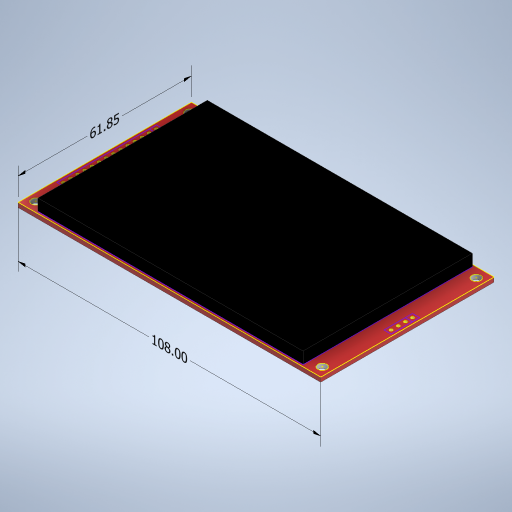
# Autodesk Inventor part: ILI9488
Saved by Autodesk Inventor 2024 (Build 280153000, 153)
## iProperties
Created: 2024-01-05
Part Number: ILI9488
Material: Genérico
Document SubType Name: Modeling
Designer: sergi
Density: 1 g/cm^3
Appearance: Valor por defecto
Author: sergi
Autodesk Inventor part; units mm, degrees
ref_plane "YZ Plane" through (0, 0, 0) normal (1, 0, 0) x (0, 1, 0)
ref_plane "XZ Plane" through (0, 0, 0) normal (0, 1, 0) x (-1, 0, 0)
ref_plane "XY Plane" through (0, 0, 0) normal (0, 0, 1) x (1, 0, 0)
sketch "Boceto1" plane through (0, 0, 0) normal (0, 1, 0) x (-1, 0, 0)
  line L0 (-54, 30.925) -> (54, 30.925)
  line L1 (54, 30.925) -> (54, -30.925)
  line L2 (54, -30.925) -> (-54, -30.925)
  line L3 (-54, -30.925) -> (-54, 30.925)
  line L4 (-54, 30.925) -> (54, -30.925) construction
  line L5 (54, 30.925) -> (-54, -30.925) construction
  line L6 (54, -30.925) -> (54, -29.075)
  circle A0 centre (-51.1, -27.475) radius 1.6
  circle A1 centre (51.1, -27.475) radius 1.6
  circle A2 centre (51.1, 27.475) radius 1.6
  circle A3 centre (-51.1, 27.475) radius 1.6
  line L7 (54, 30.925) -> (54, 29.075)
  line L8 (-50.7696, -29.075) -> (-51.1, -29.075)
  line L9 (-50.7696, 29.075) -> (-51.1, 29.075)
  line L10 (51.1, 29.075) -> (50.7696, 29.075)
  point P0 (0, 0)
  dimension "d4" = 3.2
  dimension "d6" = 3.2
  dimension "d7" = 3.2
  dimension "d0" = 108
  dimension "d1" = 61.85
  dimension "d5" = 3.2
  constraints: 22 end point, 6 horizontal, 5 point on line, 4 perpendicular, 3 vertical alignment, 2 midpoint, 2 parallel, 1 centre point, 1 tangent, 6 other
  measures "d0" distance of L1.end L2.end
  measures "d1" distance of L0.end L1.end
  measures "d5" diameter of A1
extrude "Extrusión1" add sketch "Boceto1" along normal blind 1.65
sketch "Boceto2" plane through (0, 1.65, 0) normal (0, 1, 0) x (1, 0, 0)
  line L0 (54, -30.925) -> (54, 30.925) projected
  line L1 (54, 30.925) -> (-54, 30.925) projected
  line L2 (-54, 30.925) -> (-54, -30.925) projected
  line L3 (-54, -30.925) -> (54, -30.925) projected
  circle A0 centre (51.1, 27.475) radius 1.6 projected
  circle A1 centre (-51.1, 27.475) radius 1.6 projected
  circle A2 centre (-51.1, -27.475) radius 1.6 projected
  circle A3 centre (51.1, -27.475) radius 1.6 projected
  line L4 (54, 30.925) -> (54, 5.075)
  line L5 (54, -30.925) -> (54, 30.925) projected
  line L6 (54, 5.075) -> (53.25, 5.075)
  line L7 (53.25, 5.075) -> (50.71, 5.075)
  line L8 (50.71, 5.075) -> (50.71, -5.085)
  line L9 (50.71, -5.085) -> (53.25, -5.085)
  line L10 (53.25, -5.085) -> (53.25, 5.075)
  line L11 (51.98, 5.075) -> (51.98, -5.085)
  line L12 (51.98, 5.075) -> (51.98, 3.805)
  line L13 (51.98, 3.805) -> (51.98, 1.265)
  line L14 (51.98, 1.265) -> (51.98, -1.275)
  line L15 (51.98, -1.275) -> (51.98, -3.815)
  circle A4 centre (51.98, 3.805) radius 0.5
  circle A5 centre (51.98, 1.265) radius 0.5
  circle A6 centre (51.98, -1.275) radius 0.5
  circle A7 centre (51.98, -3.815) radius 0.5
  line L16 (-54, 30.925) -> (-53.25, 30.925)
  line L17 (54, 30.925) -> (-54, 30.925) projected
  line L18 (-53.25, 30.925) -> (-53.25, 17.675)
  line L19 (-53.25, 17.675) -> (-50.71, 17.675)
  line L20 (-50.71, 17.675) -> (-50.71, -17.885)
  line L21 (-50.71, -17.885) -> (-53.25, -17.885)
  line L22 (-53.25, -17.885) -> (-53.25, 17.675)
  line L23 (-51.98, 17.675) -> (-51.98, 16.405)
  circle A8 centre (-51.98, 16.405) radius 0.5
  line L24 (-51.98, 16.405) -> (-51.98, 13.851)
  line L25 (-51.98, 15.121) -> (-51.98, 13.851)
  circle A9 centre (-51.98, 13.851) radius 0.5
  line L26 (-51.98, 13.851) -> (-51.98, 11.297)
  line L27 (-51.98, 12.567) -> (-51.98, 11.297)
  circle A10 centre (-51.98, 11.297) radius 0.5
  line L28 (-51.98, 11.297) -> (-51.98, 8.743)
  line L29 (-51.98, 8.743) -> (-51.98, 6.189)
  circle A11 centre (-51.98, 8.743) radius 0.5
  line L30 (-51.98, 6.189) -> (-51.98, 3.635)
  circle A12 centre (-51.98, 6.189) radius 0.5
  line L31 (-51.98, 3.635) -> (-51.98, 1.081)
  circle A13 centre (-51.98, 3.635) radius 0.5
  line L32 (-51.98, 1.081) -> (-51.98, -1.473)
  circle A14 centre (-51.98, 1.081) radius 0.5
  line L33 (-51.98, -1.473) -> (-51.98, -4.027)
  circle A15 centre (-51.98, -1.473) radius 0.5
  line L34 (-51.98, -4.027) -> (-51.98, -6.581)
  circle A16 centre (-51.98, -4.027) radius 0.5
  line L35 (-51.98, -6.581) -> (-51.98, -9.135)
  circle A17 centre (-51.98, -6.581) radius 0.5
  line L36 (-51.98, -9.135) -> (-51.98, -11.689)
  circle A18 centre (-51.98, -9.135) radius 0.5
  line L37 (-51.98, -11.689) -> (-51.98, -14.243)
  circle A19 centre (-51.98, -11.689) radius 0.5
  line L38 (-51.98, -14.243) -> (-51.98, -16.797)
  circle A20 centre (-51.98, -14.243) radius 0.5
  line L39 (-51.98, -16.797) -> (-51.98, -19.351)
  circle A21 centre (-51.98, -16.797) radius 0.5
  point P0 (0, 0)
  dimension "d11" = 25.85
  dimension "d12" = 0.75
  dimension "d13" = 2.54
  dimension "d14" = 10.16
  dimension "d15" = 1.27
  dimension "d16" = 2.54
  dimension "d17" = 2.54
  dimension "d18" = 2.54
  dimension "d19" = 1
  dimension "d20" = 1
  dimension "d21" = 1
  dimension "d22" = 1
  dimension "d30" = 0.75
  dimension "d31" = 13.25
  dimension "d32" = 2.54
  dimension "d33" = 35.56
  dimension "d34" = 1.27
  dimension "d35" = 1
  dimension "d36" = 2.554
  dimension "d37" = 1.27
  dimension "d38" = 1
  dimension "d39" = 2.554
  dimension "d40" = 1.27
  dimension "d41" = 1
  dimension "d42" = 2.554
  dimension "d43" = 1
  dimension "d44" = 2.554
  dimension "d45" = 1
  dimension "d46" = 2.554
  dimension "d47" = 1
  dimension "d48" = 2.554
  dimension "d49" = 1
  dimension "d50" = 2.554
  dimension "d51" = 1
  dimension "d52" = 2.554
  dimension "d53" = 1
  dimension "d54" = 2.554
  dimension "d55" = 1
  dimension "d56" = 2.554
  dimension "d57" = 1
  dimension "d58" = 2.554
  dimension "d59" = 1
  dimension "d60" = 2.554
  dimension "d61" = 1
  dimension "d62" = 2.554
  dimension "d63" = 1
  dimension "d64" = 2.554
  constraints: 68 end point, 18 centre point, 18 vertical, 7 coincident, 6 point on line, 4 parallel, 3 horizontal, 3 midpoint, 2 perpendicular
  measures "d11" distance of L0.end L4.end
  measures "d12" distance of L4.end L6.end
  measures "d13" distance of L9.end L8.end
  measures "d14" distance of L8.end L7.end
  measures "d15" distance of L11.start L12.end
  measures "d16" distance of L12.end L13.end
  measures "d17" distance of L13.end L14.end
  measures "d18" distance of L14.end L15.end
  measures "d19" diameter of A4
  measures "d20" diameter of A5
  measures "d21" diameter of A6
  measures "d22" diameter of A7
  measures "d30" distance of L1.end L16.end
  measures "d31" distance of L16.end L18.end
  measures "d32" distance of L20.end L21.end
  measures "d33" distance of L19.end L20.end
  measures "d34" distance of L23.start L23.end
  measures "d35" diameter of A8
  measures "d36" distance of L24.start L24.end
  measures "d37" distance of L25.start L25.end
  measures "d38" diameter of A9
  measures "d39" distance of L26.start L26.end
  measures "d40" distance of L27.start L27.end
  measures "d41" diameter of A10
  measures "d42" distance of L28.start L28.end
  measures "d43" diameter of A11
  measures "d44" distance of L29.start L29.end
  measures "d45" diameter of A12
  measures "d46" distance of L30.start L30.end
  measures "d47" diameter of A13
  measures "d48" distance of L31.start L31.end
  measures "d49" diameter of A14
  measures "d50" distance of L32.start L32.end
  measures "d51" diameter of A15
  measures "d52" distance of L33.start L33.end
  measures "d53" diameter of A16
  measures "d54" distance of L34.start L34.end
  measures "d55" diameter of A17
  measures "d56" distance of L35.start L35.end
  measures "d57" diameter of A18
  measures "d58" distance of L36.start L36.end
  measures "d59" diameter of A19
  measures "d60" distance of L37.start L37.end
  measures "d61" diameter of A20
  measures "d62" distance of L38.start L38.end
  measures "d63" diameter of A21
  measures "d64" distance of L39.start L39.end
hole "Agujero1" at (51.98, 1.65, -3.805) at (51.98, 1.65, -1.265) at (51.98, 1.65, 1.275) at (51.98, 1.65, 3.815) at (-51.98, 1.65, -16.405) at (-51.98, 1.65, -13.851) at (-51.98, 1.65, -11.297) at (-51.98, 1.65, -8.743) at (-51.98, 1.65, -6.189) at (-51.98, 1.65, -3.635) at (-51.98, 1.65, -1.081) at (-51.98, 1.65, 1.473) at (-51.98, 1.65, 4.027) at (-51.98, 1.65, 6.581) at (-51.98, 1.65, 9.135) at (-51.98, 1.65, 11.689) at (-51.98, 1.65, 14.243) at (-51.98, 1.65, 16.797) direction (0, -1, 0) diameter 1 end through all
sketch "Boceto3" plane through (0, 1.65, 0) normal (0, 1, 0) x (1, 0, 0)
  circle A0 centre (-51.98, -16.797) radius 0.5 projected
  circle A1 centre (-51.98, -14.243) radius 0.5 projected
  circle A2 centre (-51.98, -11.689) radius 0.5 projected
  circle A3 centre (-51.98, -9.135) radius 0.5 projected
  circle A4 centre (-51.98, -6.581) radius 0.5 projected
  circle A5 centre (-51.98, -4.027) radius 0.5 projected
  circle A6 centre (-51.98, -1.473) radius 0.5 projected
  circle A7 centre (-51.98, 1.081) radius 0.5 projected
  circle A8 centre (-51.98, 3.635) radius 0.5 projected
  circle A9 centre (-51.98, 6.189) radius 0.5 projected
  circle A10 centre (-51.98, 8.743) radius 0.5 projected
  circle A11 centre (-51.98, 11.297) radius 0.5 projected
  circle A12 centre (-51.98, 13.851) radius 0.5 projected
  circle A13 centre (-51.98, 16.405) radius 0.5 projected
  circle A14 centre (51.98, -3.815) radius 0.5 projected
  circle A15 centre (51.98, -1.275) radius 0.5 projected
  circle A16 centre (51.98, 1.265) radius 0.5 projected
  circle A17 centre (51.98, 3.805) radius 0.5 projected
  line L0 (54, -30.925) -> (54, 30.925) projected
  line L1 (54, 30.925) -> (-54, 30.925) projected
  line L2 (-54, 30.925) -> (-54, -30.925) projected
  line L3 (-54, -30.925) -> (54, -30.925) projected
  circle A18 centre (51.1, 27.475) radius 1.6 projected
  circle A19 centre (-51.1, 27.475) radius 1.6 projected
  circle A20 centre (-51.1, -27.475) radius 1.6 projected
  circle A21 centre (51.1, -27.475) radius 1.6 projected
  line L4 (-51.98, 17.675) -> (-50.71, 17.675)
  line L5 (-50.71, 17.675) -> (-53.25, 17.675)
  line L6 (-53.25, 17.675) -> (-53.25, -17.885)
  line L7 (-53.25, -17.885) -> (-50.71, -17.885)
  line L8 (-50.71, -17.885) -> (-50.71, 17.675)
  line L9 (-53.25, 17.675) -> (-53.25, 15.135)
  line L10 (-53.25, 15.135) -> (-50.71, 15.135)
  line L11 (51.98, 5.075) -> (53.25, 5.075)
  line L12 (53.25, 5.075) -> (50.71, 5.075)
  line L13 (50.71, 5.075) -> (50.71, -5.085)
  line L14 (50.71, -5.085) -> (53.25, -5.085)
  line L15 (53.25, -5.085) -> (53.25, 5.075)
  line L16 (50.71, -5.085) -> (50.71, -4.818)
  line L17 (50.71, 5.075) -> (50.71, 2.535)
  line L18 (50.71, 2.535) -> (53.25, 2.535)
  line L19 (54, 30.925) -> (-54, 30.925) projected
  line L20 (-47.6, 30.225) -> (47, 30.225)
  line L21 (47, 30.225) -> (47, -30.225)
  line L22 (47, -30.225) -> (-47.6, -30.225)
  line L23 (-47.6, -30.225) -> (-47.6, 30.225)
  point P0 (0, 0)
  constraints: 38 end point, 6 parallel, 6 perpendicular, 5 point on line, 3 horizontal
sketch "Boceto4" plane through (0, 1.65, 0) normal (0, 1, 0) x (1, 0, 0)
  line L0 (-47.6, -30.225) -> (-47.6, 30.225) projected
  line L1 (47, 30.225) -> (47, -30.225) projected
  line L2 (-47.6, 30.225) -> (47, 30.225) projected
  line L3 (47, -30.225) -> (-47.6, -30.225) projected
  point P0 (0, 0)
extrude "Extrusión2" add sketch "Boceto4" along normal blind 4.15
sketch "Boceto5" plane through (0, 0, 0) normal (0, -1, 0) x (1, 0, 0)
  circle A0 centre (-51.98, 16.797) radius 0.5 projected
  circle A1 centre (-51.98, 14.243) radius 0.5 projected
  circle A2 centre (-51.98, 11.689) radius 0.5 projected
  circle A3 centre (-51.98, 9.135) radius 0.5 projected
  circle A4 centre (-51.98, 6.581) radius 0.5 projected
  circle A5 centre (-51.98, 4.027) radius 0.5 projected
  circle A6 centre (-51.98, 1.473) radius 0.5 projected
  circle A7 centre (-51.98, -1.081) radius 0.5 projected
  circle A8 centre (-51.98, -3.635) radius 0.5 projected
  circle A9 centre (-51.98, -6.189) radius 0.5 projected
  circle A10 centre (-51.98, -8.743) radius 0.5 projected
  circle A11 centre (-51.98, -11.297) radius 0.5 projected
  circle A12 centre (-51.98, -13.851) radius 0.5 projected
  circle A13 centre (-51.98, -16.405) radius 0.5 projected
  circle A14 centre (51.98, 3.815) radius 0.5 projected
  circle A15 centre (51.98, 1.275) radius 0.5 projected
  circle A16 centre (51.98, -1.265) radius 0.5 projected
  circle A17 centre (51.98, -3.805) radius 0.5 projected
  line L0 (54, 30.925) -> (54, -30.925) projected
  line L1 (-54, 30.925) -> (54, 30.925) projected
  line L2 (-54, -30.925) -> (-54, 30.925) projected
  line L3 (54, -30.925) -> (-54, -30.925) projected
  circle A18 centre (51.1, -27.475) radius 1.6 projected
  circle A19 centre (-51.1, -27.475) radius 1.6 projected
  circle A20 centre (-51.1, 27.475) radius 1.6 projected
  circle A21 centre (51.1, 27.475) radius 1.6 projected
  line L4 (54, -30.925) -> (45.6, -30.925)
  line L5 (45.6, -30.925) -> (19.1, -30.925)
  line L6 (19.1, -30.925) -> (19.1, -10.525)
  line L7 (19.1, -10.525) -> (45.6, -10.525)
  line L8 (45.6, -10.525) -> (45.6, -30.925)
  line L9 (45.6, -30.925) -> (45.6, -29.925)
  line L10 (45.6, -29.925) -> (19.1, -29.925)
  point P0 (0, 0)
  dimension "d81" = 8.4
  dimension "d82" = 26.5
  dimension "d83" = 20.4
  dimension "d86" = 1
  constraints: 14 end point, 3 point on line, 2 parallel, 2 perpendicular, 1 horizontal
  measures "d81" distance of L0.end L4.end
  measures "d82" distance of L6.end L7.end
  measures "d83" distance of L5.end L6.end
  measures "d86" distance of L4.end L9.end
extrude "Extrusión3" add sketch "Boceto5" along normal blind 3 contours L10 L6 L7 L8
